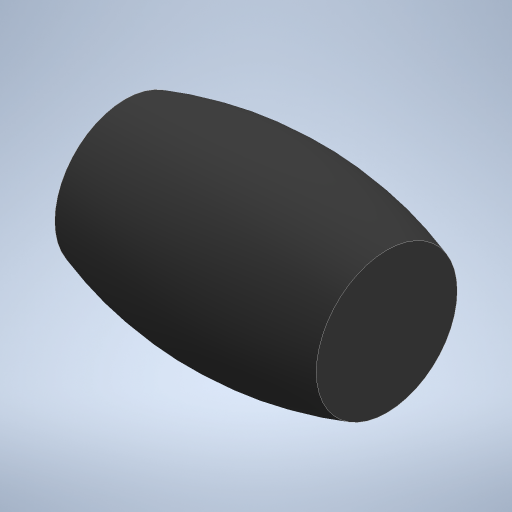
# Autodesk Inventor part: ballel
Saved by Autodesk Inventor 2024.1 (Build 281209000, 209)
## iProperties
Created: 2024-11-26
Part Number: ballel
Material: ゴム
Document SubType Name: Modeling
Designer: hibik
Density: 0.93 g/cm^3
Appearance: ゴム - 黒
Author: hibik
Autodesk Inventor part; units mm, degrees
ref_plane "YZ Plane" through (0, 0, 0) normal (1, 0, 0) x (0, 1, 0)
ref_plane "XZ Plane" through (0, 0, 0) normal (0, 1, 0) x (-1, 0, 0)
ref_plane "XY Plane" through (0, 0, 0) normal (0, 0, 1) x (1, 0, 0)
sketch "スケッチ1" plane through (0, 0, 0) normal (0, 0, 1) x (1, 0, 0)
  circle A0 centre (0, -22.5) radius 29
  line L0 (-9.25, 6.5) -> (9.25, 6.5)
  line L1 (9.25, 6.5) -> (9.25, -22.5)
  line L2 (9.25, -22.5) -> (-9.25, -22.5)
  line L3 (-9.25, -22.5) -> (-9.25, 6.5)
  line L4 (-9.25, 0) -> (9.25, 0)
  point P0 (9.25, 4.9852)
  point P1 (-9.25, 4.9852)
  point P2 (0, 0)
  dimension "d0" = 58
  dimension "d1" = 18.5
  dimension "d2" = 6.5
  constraints: 10 end point, 2 coincident, 2 midpoint, 2 parallel, 2 perpendicular, 2 point on line, 1 centre point, 1 horizontal, 1 tangent, 1 vertical alignment
  measures "d0" diameter of A0
  measures "d1" distance of L0.start L0.end
  measures "d2" distance between parallel lines of L0 L4
revolve "回転1" add sketch "スケッチ1" angle 360 about axis through (-9.25, 0, 0) along (1, 0, 0) contours L1 L4 L3 A0
